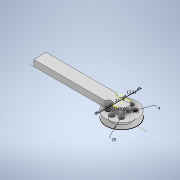
# Autodesk Inventor part: US holder1
Saved by Autodesk Inventor 2022 (Build 260153000, 153)
## iProperties
Created: 2022-07-18
Part Number: US holder1
Material: Generic
Document SubType Name: Modeling
Designer: biom
Density: 1 g/cm^3
Appearance: Default
Author: biom
Autodesk Inventor part; units mm, degrees
ref_plane "YZ Plane" through (0, 0, 0) normal (1, 0, 0) x (0, 1, 0)
ref_plane "XZ Plane" through (0, 0, 0) normal (0, 1, 0) x (-1, 0, 0)
ref_plane "XY Plane" through (0, 0, 0) normal (0, 0, 1) x (1, 0, 0)
sketch "Sketch1" plane through (0, 0, 0) normal (0, 1, 0) x (-1, 0, 0)
  circle A0 centre (0, 0) radius 12.5
  line L0 (0, 0) -> (7.75, 0) construction
  circle A1 centre (5.4801, -5.4801) radius 2
  circle A2 centre (-5.4801, -5.4801) radius 2
  circle A3 centre (-5.4801, 5.4801) radius 2
  circle A4 centre (5.4801, 5.4801) radius 2
  circle A5 centre (0, -7.75) radius 2
  circle A6 centre (0, 7.75) radius 2
  dimension "d0" = 25
  dimension "d3" = 4
  dimension "d6" = 360
  dimension "d8" = 4
  dimension "d11" = 360
  constraints: 7 centre point, 3 coincident, 2 end point, 1 horizontal, 16 other
  measures "d0" diameter of A0
  measures "d3" diameter of A1
  measures "d8" diameter of A5
extrude "Extrusion1" add sketch "Sketch1" along normal blind 5
sketch "Sketch2" plane through (0, 5, 0) normal (0, 1, 0) x (1, 0, 0)
  line L0 (4.991, -3.5408) -> (4.991, 3.5408)
  line L1 (-66.4503, 5) -> (-66.4503, -5)
  line L2 (4.991, -4.9385) -> (14.991, -4.9385) construction
  line L3 (-82.7386, 0) -> (31.2793, 0) projected
  arc A0 (-3.5548, -4.9385) -> (-7.4216, -5) centre (-5.4801, -5.4801) ccw
  line L4 (-66.4503, -5) -> (-7.4216, -5)
  line L5 (-3.5548, -4.9385) -> (3.5548, -4.9385)
  circle A1 centre (-5.4801, 5.4801) radius 2 projected
  arc A2 (-7.4216, 5) -> (-3.5497, 4.9571) centre (-5.4801, 5.4801) ccw
  line L6 (3.5497, 4.9571) -> (-3.5497, 4.9571)
  line L7 (-7.4216, 5) -> (-66.4503, 5)
  arc A3 (4.991, -3.5408) -> (3.5548, -4.9385) centre (5.4801, -5.4801) ccw
  circle A4 centre (5.4801, 5.4801) radius 2 projected
  arc A5 (3.5497, 4.9571) -> (4.991, 3.5408) centre (5.4801, 5.4801) ccw
  dimension "d24" = 10
  dimension "d25" = 90
  dimension "d26" = 70
  dimension "d27" = 4
  dimension "d28" = 4
  dimension "d29" = 4
  dimension "d30" = 4
  constraints: 14 end point, 8 point on circle, 7 parallel, 4 centre point, 4 coincident, 2 perpendicular, 1 horizontal, 1 vertical
  measures "d24" distance of L2.start L6.start
  measures "d25" angle of L2 L0
  measures "d26" distance of L1.start L6.start
  measures "d27" diameter of A0
  measures "d28" diameter of A2
  measures "d29" diameter of A3
  measures "d30" diameter of A5
extrude "Extrusion2" add sketch "Sketch2" along normal blind 5 contours A3 L5 A0 L4 L1 L3 L0 | L3 L1 L7 A1 L6 A4 L0
sketch "Sketch4" plane through (0, 10, 0) normal (0, 1, 0) x (1, 0, 0)
  line L0 (-3.5548, -4.9385) -> (3.5548, -4.9385) projected
  line L1 (-3.5548, -4.9385) -> (3.5548, -4.9385)
  line L2 (3.5497, 4.9571) -> (-3.5497, 4.9571) projected
  line L3 (-3.5497, 4.9571) -> (3.5497, 4.9571)
  line L4 (-4.4956, -10.2074) -> (2.6201, -10.2074)
  point P0 (0, 0)
  constraints: 6 end point, 3 horizontal
sketch "Sketch8" plane through (0, 5, 0) normal (0, 1, 0) x (1, 0, 0)
  circle A0 centre (-5.4801, 5.4801) radius 2 projected
  circle A1 centre (-5.4801, 5.4801) radius 3
  circle A2 centre (-5.4801, -5.4801) radius 2 projected
  circle A3 centre (-5.4801, -5.4801) radius 3
  circle A4 centre (5.4801, 5.4801) radius 2 projected
  circle A5 centre (5.4801, 5.4801) radius 3
  arc A6 (3.5548, -4.9385) -> (4.991, -3.5408) centre (5.4801, -5.4801) ccw projected
  circle A7 centre (5.4801, -5.4801) radius 3
  point P0 (0, 0)
  dimension "d50" = 6
  dimension "d51" = 6
  dimension "d52" = 6
  dimension "d53" = 6
  constraints: 4 centre point, 4 coincident
  measures "d50" diameter of A1
  measures "d51" diameter of A3
  measures "d52" diameter of A5
  measures "d53" diameter of A7
extrude "Extrusion6" cut sketch "Sketch8" along normal blind 39.25 contours A0 | A1 | A2 | A3 | A4 | A5 | A7
sketch "Sketch33" plane through (0, 10, 0) normal (0, 1, 0) x (1, 0, 0)
  line L0 (-2.5294, -4.9385) -> (2.5294, -4.9385) projected
  arc A0 (-8.4414, 5) -> (-2.526, 4.9571) centre (-5.4801, 5.4801) ccw projected
  line L1 (-2.5294, -4.9385) -> (-2.526, 4.9571)
  line L2 (-2.526, 4.9571) -> (-2.526, 4.9571)
  line L3 (2.526, 4.9571) -> (-2.526, 4.9571) projected
  line L4 (-2.526, 4.9571) -> (-2.5215, 18.4671)
  line L5 (-2.5215, 18.4671) -> (-2.534, -18.5329)
  point P0 (0, 0)
  dimension "d105" = 13.51
  dimension "d106" = 37
  constraints: 8 end point, 2 point on line
  measures "d105" distance of L1.end L4.end
  measures "d106" distance of L4.end L5.end
sketch "Sketch34" plane through (-66.4503, 5, -5) normal (-1, 0, 0) x (0, 0, 1)
  point P0 (5, -5)
body "Solid1"
